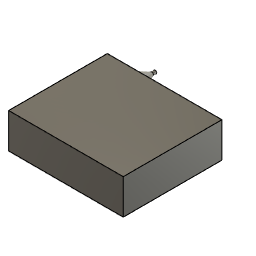
Ladekoffer (Autodesk Fusion 360 archive; units mm, degrees)
design "Netzteil"
Autodesk Fusion 360 part; units mm, degrees
sketch "Skizze1" plane through (0, 0, 0) normal (0, 0, 1) x (1, 0, 0)
  line L0 (-90, 27.5) -> (90, 27.5)
  line L1 (90, 27.5) -> (90, -27.5)
  line L2 (90, -27.5) -> (-90, -27.5)
  line L3 (-90, -27.5) -> (-90, 27.5)
  line L4 (-90, 27.5) -> (90, -27.5) construction
  line L5 (90, 27.5) -> (-90, -27.5) construction
  dimension "d1" = 180
  dimension "d2" = 55
  constraint horizontal L0
  constraint perpendicular L0 L1
  constraint parallel L0 L2
  constraint parallel L1 L3
  constraint coincident L4 origin
  constraint coincident L5 origin
  measures "d1" distance of L1.end L2.end
  measures "d2" distance of L0.end L1.end
extrude "Extrusion1" add sketch "Skizze1" along normal mid plane 155
sketch "Skizze3" plane through (0, 0, 0) normal (0, 1, 0) x (1, 0, 0)
  line L0 (90, 77.5) -> (-90, 77.5)
  line L1 (-90, 77.5) -> (90, 77.5)
  line L2 (-70, 77.5) -> (-70, 87.5)
  line L3 (-70, 87.5) -> (-55, 87.5)
  line L4 (-55, 77.5) -> (-55, 117.5)
  line L5 (-55, 117.5) -> (-57.5, 117.5)
  line L6 (-57.5, 117.5) -> (-57.5, 112.5)
  line L7 (-57.5, 112.5) -> (-70, 87.5)
  dimension "d5" = 10
  dimension "d6" = 15
  dimension "d7" = 2.5
  dimension "d8" = 5
  dimension "d9" = 40
  dimension "d10" = 20
  constraint coincident L1 L2.start
  constraint perpendicular L0 L2
  constraint perpendicular L2 L3
  constraint coincident L0 L4.start
  constraint perpendicular L0 L4
  constraint perpendicular L4 L5
  constraint perpendicular L5 L6
  constraint coincident L3.end L4
  measures "d5" distance of L2.start L2.end
  measures "d6" distance of L2.end L3.end
  measures "d7" distance of L4.end L5.end
  measures "d8" distance of L5.end L6.end
  measures "d9" distance of L4.start L4.end
  measures "d10" distance of L0.end L2.start
revolve "Drehen1" add sketch "Skizze3" angle 360 about axis through (-55, 0, -77.5) along (0, 0, -1)

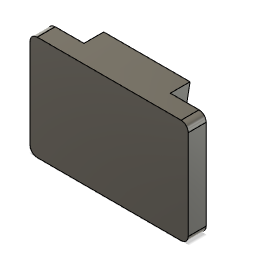
design "ISDT SC608"
Autodesk Fusion 360 part; units mm, degrees
sketch "Skizze1" plane through (0, 0, 0) normal (0, 0, 1) x (1, 0, 0)
  line L0 (-44, 29) -> (44, 29)
  line L1 (44, 29) -> (44, -29)
  line L2 (44, -29) -> (-44, -29)
  line L3 (-44, -29) -> (-44, 29)
  line L4 (-44, 29) -> (44, -29) construction
  line L5 (44, 29) -> (-44, -29) construction
  dimension "d1" = 88
  dimension "d2" = 58
  constraint horizontal L0
  constraint perpendicular L0 L1
  constraint parallel L0 L2
  constraint parallel L1 L3
  constraint coincident L4 origin
  constraint coincident L5 origin
  measures "d1" distance of L1.end L2.end
  measures "d2" distance of L0.end L1.end
extrude "Extrusion1" add sketch "Skizze1" along normal blind 21
sketch "Skizze2" plane through (44, 0, 0) normal (1, 0, 0) x (0, 0, -1)
  line L0 (0, -29) -> (0, 29)
  line L1 (0, 29) -> (-21, 29)
  line L2 (-21, 29) -> (-21, -29)
  line L3 (-21, -29) -> (0, -29)
  line L4 (-11, -29) -> (0, 29)
  dimension "d5" = 10
  constraint coincident L0.end L1.start
  constraint coincident L3 L4.start
  measures "d5" distance of L2 L4.start
extrude "Extrusion2" cut sketch "Skizze2" against normal blind 91 contours L0 L3 L4
sketch "Skizze3" plane through (44, 0, 0) normal (1, 0, 0) x (0, 0, -1)
  line L0 (-11, -29) -> (0, 29)
  line L1 (0, 29) -> (-21, 29)
  line L2 (-21, 29) -> (-21, -29)
  line L3 (-21, -29) -> (-11, -29)
  line L4 (-11, -29) -> (-11, 29.0011)
  constraint coincident L0.start L3.end
  constraint vertical L4
extrude "Extrusion3" cut sketch "Skizze3" against normal blind 20 contours L0 L1 L4
sketch "Skizze4" plane through (-44, 0, 0) normal (-1, 0, 0) x (0, 0, 1)
  line L0 (0, 29) -> (11, -29)
  line L1 (11, -29) -> (21, -29)
  line L2 (21, -29) -> (21, 29)
  line L3 (21, 29) -> (0, 29)
  line L4 (11, -29) -> (11, 29)
  constraint coincident L0.end L1.start
  constraint coincident L3 L4.end
  constraint vertical L4
extrude "Extrusion4" cut sketch "Skizze4" against normal blind 20 contours L0 L3 L4
fillet "Abrundung1" radius 4 4 edges at (-44, 29, 16) (-44, -29, 16) (44, -29, 16) (44, 29, 16)

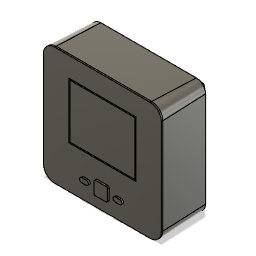
design "ISDT P20"
Autodesk Fusion 360 part; units mm, degrees
sketch "Skizze1" plane through (0, 0, 0) normal (0, 0, 1) x (1, 0, 0)
  line L0 (52.75, 52.75) -> (-52.75, 52.75)
  line L1 (-52.75, 52.75) -> (-52.75, -52.75)
  line L2 (-52.75, -52.75) -> (52.75, -52.75)
  line L3 (52.75, -52.75) -> (52.75, 52.75)
  line L4 (52.75, 52.75) -> (-52.75, -52.75) construction
  line L5 (-52.75, 52.75) -> (52.75, -52.75) construction
  dimension "d1" = 105.5
  constraint horizontal L0
  constraint perpendicular L0 L1
  constraint parallel L0 L2
  constraint parallel L1 L3
  constraint coincident L4 origin
  constraint coincident L5 origin
  constraint equal L0 L1
  measures "d1" distance of L0.end L1.end
extrude "Extrusion1" add sketch "Skizze1" along normal blind 47.3
fillet "Abrundung1" radius 10 4 edges at (-52.75, -52.75, 23.65) (52.75, -52.75, 23.65) (52.75, 52.75, 23.65) (-52.75, 52.75, 23.65)
chamfer "Fase1" distance 46 distance2 2 8 edges at (0, -52.75, 0) (49.8211, -49.8211, 0) (52.75, 0, 0) (49.8211, 49.8211, 0) (0, 52.75, 0) (-49.8211, 49.8211, 0) (-52.75, 0, 0) (-49.8211, -49.8211, 0) measured on face at (-14.25, -52.75, 15.7667) measured on face at (43.2258, -52.7387, 15.7667) measured on face at (52.75, -14.25, 15.7667) measured on face at (43.2258, 52.7387, 15.7667) measured on face at (14.25, 52.75, 15.7667) measured on face at (-43.2258, 52.7387, 15.7667) measured on face at (-52.75, 14.25, 15.7667) measured on face at (-43.7006, -52.7047, 15.7667)
chamfer "Fase2" distance 6 distance2 7 8 edges at (50.75, 0, 0) (48.4069, 48.4069, 0) (0, 50.75, 0) (-48.4069, 48.4069, 0) (-50.75, 0, 0) (-48.4069, -48.4069, 0) (0, -50.75, 0) (48.4069, -48.4069, 0) measured on face at (52.0833, -14.25, 30.6667) measured on face at (43.5386, 51.7632, 24.0952) measured on face at (14.25, 51.4167, 15.3333) measured on face at (-51.7632, 43.5386, 24.0952) measured on face at (-52.0833, 14.25, 30.6667) measured on face at (-43.5386, -51.7632, 24.0952) measured on face at (-14.25, -51.4167, 15.3333) measured on face at (51.7632, -43.5386, 24.0952)
sketch "Skizze2" plane through (0, 0, 47.3) normal (0, 0, 1) x (1, 0, 0)
  arc A0 (-42.75, 52.75) -> (-52.75, 42.75) centre (-42.75, 42.75) ccw
  line L0 (-52.75, 42.75) -> (-52.75, -42.75)
  arc A1 (-52.75, -42.75) -> (-42.75, -52.75) centre (-42.75, -42.75) ccw
  line L1 (-42.75, -52.75) -> (42.75, -52.75)
  arc A2 (42.75, -52.75) -> (52.75, -42.75) centre (42.75, -42.75) ccw
  line L2 (52.75, -42.75) -> (52.75, 42.75)
  arc A3 (52.75, 42.75) -> (42.75, 52.75) centre (42.75, 42.75) ccw
  line L3 (42.75, 52.75) -> (-42.75, 52.75)
  line L4 (6, -42.75) -> (-6, -42.75)
  line L5 (-6, -42.75) -> (-6, -30.75)
  line L6 (-6, -30.75) -> (6, -30.75)
  line L7 (6, -30.75) -> (6, -42.75)
  line L8 (6, -42.75) -> (-6, -30.75) construction
  line L9 (-6, -42.75) -> (6, -30.75) construction
  line L10 (-19, -34.75) -> (-11, -34.75)
  line L11 (-11, -34.75) -> (-11, -38.75)
  line L12 (-11, -38.75) -> (-19, -38.75)
  line L13 (-19, -38.75) -> (-19, -34.75)
  line L14 (-19, -34.75) -> (-11, -38.75) construction
  line L15 (-11, -34.75) -> (-19, -38.75) construction
  line L16 (0, -36.75) -> (0, -42.75) construction
  line L17 (19, -34.75) -> (11, -38.75) construction
  line L18 (11, -34.75) -> (11, -38.75)
  line L19 (19, -38.75) -> (19, -34.75)
  line L20 (11, -34.75) -> (19, -38.75) construction
  line L21 (19, -34.75) -> (11, -34.75)
  line L22 (11, -38.75) -> (19, -38.75)
  point P0 (0, -36.75)
  point P1 (-15, -36.75)
  point P2 (15, -36.75)
  dimension "d10" = 12
  dimension "d11" = 12
  dimension "d12" = 8
  dimension "d13" = 4
  dimension "d14" = 10
  dimension "d15" = 5
  constraint horizontal L4
  constraint perpendicular L4 L5
  constraint parallel L4 L6
  constraint parallel L5 L7
  constraint coincident L8 P0
  constraint coincident L9 P0
  constraint horizontal L10
  constraint perpendicular L10 L11
  constraint parallel L10 L12
  constraint parallel L11 L13
  constraint coincident L14 P1
  constraint coincident L15 P1
  constraint coincident P0 L16.start
  constraint midpoint L4 L16.end
  constraint symmetric L10.start L16 L17.start
  constraint symmetric L10.end L16 L18.start
  constraint symmetric L11.end L16 L17.end
  constraint symmetric L12.end L16 L19.start
  constraint symmetric P1 L16 P2
  constraint vertical origin L16.start
  constraint horizontal P0 P1
  measures "d10" distance of L5.end L6.end
  measures "d11" distance of L4.end L5.end
  measures "d12" distance of L11.end L12.end
  measures "d13" distance of L10.end L11.end
  measures "d14" distance of L1 L16.end
  measures "d15" distance of L5 L11
extrude "Extrusion2" add sketch "Skizze2" along normal blind 1.5 contours L4 L5 L6 L7 | L10 L11 L12 L13 | L18 L19 L21 L22
fillet "Abrundung2" radius 2 8 edges at (-19, -38.75, 48.05) (-19, -34.75, 48.05) (-11, -38.75, 48.05) (-11, -34.75, 48.05) (11, -34.75, 48.05) (11, -38.75, 48.05) (19, -38.75, 48.05) (19, -34.75, 48.05)
fillet "Abrundung3" radius 1 4 edges at (-6, -42.75, 48.05) (-6, -30.75, 48.05) (6, -42.75, 48.05) (6, -30.75, 48.05)
sketch "Skizze3" plane through (0, 0, 47.3) normal (0, 0, 1) x (1, 0, 0)
  arc A0 (13, -34.75) -> (13, -38.75) centre (13, -36.75) ccw
  line L0 (13, -34.75) -> (17, -34.75)
  arc A1 (17, -38.75) -> (17, -34.75) centre (17, -36.75) ccw
  line L1 (17, -38.75) -> (13, -38.75)
  line L2 (6, -31.75) -> (6, -41.75)
  arc A2 (5, -42.75) -> (6, -41.75) centre (5, -41.75) ccw
  line L3 (5, -42.75) -> (-5, -42.75)
  arc A3 (-6, -41.75) -> (-5, -42.75) centre (-5, -41.75) ccw
  line L4 (-6, -41.75) -> (-6, -31.75)
  arc A4 (-5, -30.75) -> (-6, -31.75) centre (-5, -31.75) ccw
  line L5 (-5, -30.75) -> (5, -30.75)
  arc A5 (6, -31.75) -> (5, -30.75) centre (5, -31.75) ccw
  line L6 (-17, -34.75) -> (-13, -34.75)
  arc A6 (-13, -38.75) -> (-13, -34.75) centre (-13, -36.75) ccw
  line L7 (-13, -38.75) -> (-17, -38.75)
  arc A7 (-17, -34.75) -> (-17, -38.75) centre (-17, -36.75) ccw
  arc A8 (-42.75, 52.75) -> (-52.75, 42.75) centre (-42.75, 42.75) ccw
  line L8 (-52.75, 42.75) -> (-52.75, -42.75)
  arc A9 (-52.75, -42.75) -> (-42.75, -52.75) centre (-42.75, -42.75) ccw
  line L9 (-42.75, -52.75) -> (42.75, -52.75)
  arc A10 (42.75, -52.75) -> (52.75, -42.75) centre (42.75, -42.75) ccw
  line L10 (52.75, -42.75) -> (52.75, 42.75)
  arc A11 (52.75, 42.75) -> (42.75, 52.75) centre (42.75, 42.75) ccw
  line L11 (42.75, 52.75) -> (-42.75, 52.75)
  line L12 (30, -15) -> (-30, -15)
  line L13 (-30, -15) -> (-30, 35)
  line L14 (-30, 35) -> (30, 35)
  line L15 (30, 35) -> (30, -15)
  line L16 (30, -15) -> (-30, 35) construction
  line L17 (-30, -15) -> (30, 35) construction
  line L18 (29, -14) -> (-29, -14)
  line L19 (-29, -14) -> (-29, 34)
  line L20 (-29, 34) -> (29, 34)
  line L21 (29, 34) -> (29, -14)
  point P0 (0, 10)
  dimension "d22" = 60
  dimension "d23" = 50
  dimension "d24" = 10
  dimension "d25" = 1
  constraint horizontal L12
  constraint perpendicular L12 L13
  constraint parallel L12 L14
  constraint parallel L13 L15
  constraint coincident L16 P0
  constraint coincident L17 P0
  constraint vertical origin P0
  measures "d22" distance of L13.end L14.end
  measures "d23" distance of L12.start L14.end
  measures "d24" distance of origin P0
extrude "Extrusion3" cut sketch "Skizze3" against normal blind 1 contours L12 L13 L14 L15
